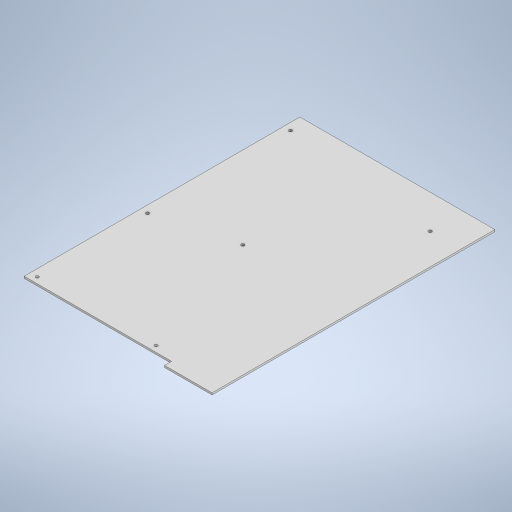
# Autodesk Inventor part: base_main_pcb
Saved by Autodesk Inventor 2024 (Build 280153000, 153)
## iProperties
Created: 2026-03-21
Part Number: base_main_pcb
Material: Generic
Document SubType Name: Modeling
Designer: schar
Density: 1 g/cm^3
Appearance: Default
Author: schar
Autodesk Inventor part; units mm, degrees
ref_plane "YZ Plane" through (0, 0, 0) normal (1, 0, 0) x (0, 1, 0)
ref_plane "XZ Plane" through (0, 0, 0) normal (0, 1, 0) x (-1, 0, 0)
ref_plane "XY Plane" through (0, 0, 0) normal (0, 0, 1) x (1, 0, 0)
sketch "Sketch1" plane through (0, 0, 0) normal (0, 1, 0) x (-1, 0, 0)
  line L0 (0, 0) -> (205, 0)
  line L1 (205, 0) -> (205, 290)
  line L2 (205, 290) -> (0, 290)
  line L3 (0, 290) -> (0, 0)
  line L4 (0, 290) -> (50, 290)
  line L5 (50, 290) -> (50, 297.4)
  line L6 (50, 297.4) -> (0, 297.4)
  line L7 (0, 297.4) -> (0, 290)
  line L8 (205, 0) -> (197.5, 0)
  line L9 (197.5, 0) -> (197.5, 17.325)
  circle A0 centre (197.5, 17.325) radius 1.675
  line L10 (197.5, 17.325) -> (197.5, 154.225)
  line L11 (197.5, 154.225) -> (197.5, 167.775)
  circle A1 centre (197.5, 167.775) radius 1.675
  line L12 (197.5, 167.775) -> (197.5, 283.785)
  circle A2 centre (197.5, 283.785) radius 1.675
  line L13 (197.5, 167.775) -> (197.5, 146.525)
  line L14 (197.5, 146.525) -> (118.5, 146.525)
  circle A3 centre (118.5, 146.525) radius 1.675
  line L15 (197.5, 283.785) -> (72.5, 283.785)
  circle A4 centre (72.5, 283.785) radius 1.675
  line L16 (197.5, 17.325) -> (197.5, 38.875)
  line L17 (197.5, 38.875) -> (32.5, 38.875)
  line L18 (32.5, 38.875) -> (32.5, 35.525)
  circle A5 centre (32.5, 35.525) radius 1.675
  dimension "d0" = 205
  dimension "d1" = 290
  dimension "d2" = 50
  dimension "d3" = 7.4
  dimension "d4" = 7.5
  dimension "d5" = 17.325
  dimension "d6" = 3.35
  dimension "d7" = 136.9
  dimension "d8" = 13.55
  dimension "d9" = 3.35
  dimension "d10" = 116.01
  dimension "d11" = 3.35
  dimension "d12" = 21.25
  dimension "d13" = 79
  dimension "d14" = 3.35
  dimension "d15" = 125
  dimension "d16" = 3.35
  dimension "d17" = 21.55
  dimension "d18" = 165
  dimension "d24" = 3.35
  constraints: 38 end point, 7 coincident, 6 centre point, 5 perpendicular, 5 point on line, 4 parallel, 3 horizontal, 2 vertical
  measures "d0" distance of L2.end L1.end
  measures "d1" distance of L1.end L0.end
  measures "d2" distance of L6.end L5.end
  measures "d3" distance of L5.end L4.end
  measures "d4" distance of L0.end L8.end
  measures "d5" distance of L8.end L9.end
  measures "d6" diameter of A0
  measures "d7" distance of L10.start L10.end
  measures "d8" distance of L10.end L11.end
  measures "d9" diameter of A1
  measures "d10" distance of L12.start L12.end
  measures "d11" diameter of A2
  measures "d12" distance of L12.start L13.end
  measures "d13" distance of L13.end L14.end
  measures "d14" diameter of A3
  measures "d15" distance of L15.start L15.end
  measures "d16" diameter of A4
  measures "d17" distance of L10.start L16.end
  measures "d18" distance of L16.end L17.end
  measures "d24" distance of L18.start L18.end
extrude "Extrusion2" add sketch "Sketch1" along normal blind 2
body "Solid2"
